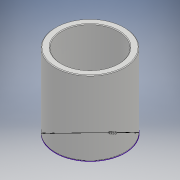
# Autodesk Inventor part: 55mmx5mm Aluminium pipe(6060)
Saved by Autodesk Inventor 2018 (Build 220112000, 112)
## iProperties
Created: 2018-03-27
Part Number: 55mmx5mm Aluminium pipe(6060)
Material: Generic
Document SubType Name: Modeling
Designer: P241310
Density: 1 g/cm^3
Appearance: Default
Author: P241310
Autodesk Inventor part; units mm, degrees
ref_plane "YZ Plane" through (0, 0, 0) normal (1, 0, 0) x (0, 1, 0)
ref_plane "XZ Plane" through (0, 0, 0) normal (0, 1, 0) x (-1, 0, 0)
ref_plane "XY Plane" through (0, 0, 0) normal (0, 0, 1) x (1, 0, 0)
sketch "Sketch1" plane through (0, 0, 0) normal (0, 0, 1) x (1, 0, 0)
  circle A0 centre (0, 0) radius 27.5
  circle A1 centre (0, 0) radius 22.5
  dimension "d0" = 55
  dimension "d1" = 45
  constraints: 2 centre point, 2 coincident
  measures "d0" diameter of A0
  measures "d1" diameter of A1
extrude "Extrusion1" add sketch "Sketch1" along normal blind 59
chamfer "Chamfer1" distance 0.5 angle 45 4 edges at (-27.5, 0, 59) (-22.5, 0, 59) (-27.5, 0, 0) (-22.5, 0, 0)
body "Solid1"
